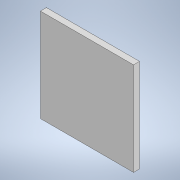
# Autodesk Inventor part: enclosure_front_plate
Saved by Autodesk Inventor 2020.2 (Build 242310000, 310)
## iProperties
Created: 2020-09-26
Part Number: enclosure_front_plate
Material: Generic
Document SubType Name: Modeling
Designer: Krishna Makhija
Density: 1 g/cm^3
Appearance: Default
Author: Krishna Makhija
Autodesk Inventor part; units mm, degrees
ref_plane "YZ Plane" through (0, 0, 0) normal (1, 0, 0) x (0, 1, 0)
ref_plane "XZ Plane" through (0, 0, 0) normal (0, 1, 0) x (-1, 0, 0)
ref_plane "XY Plane" through (0, 0, 0) normal (0, 0, 1) x (1, 0, 0)
sketch "Sketch1" plane through (0, 0, 0) normal (0, 0, 1) x (1, 0, 0)
  point P0 (0, 0)
sketch "Sketch2" plane through (0, 0, 0) normal (0, 0, 1) x (1, 0, 0)
  line L0 (-12.4002, 12.4) -> (12.4002, 12.4)
  line L1 (12.4002, 12.4) -> (12.4002, -12.4)
  line L2 (12.4002, -12.4) -> (-12.4002, -12.4)
  line L3 (-12.4002, -12.4) -> (-12.4002, 12.4)
  line L4 (-12.4002, 12.4) -> (12.4002, -12.4) construction
  line L5 (12.4002, 12.4) -> (-12.4002, -12.4) construction
  point P0 (0, 0)
  constraints: 12 end point, 2 midpoint, 2 parallel, 1 horizontal, 1 perpendicular
extrude "Extrusion1" add sketch "Sketch2" along normal blind 1.6
body "Solid1"
